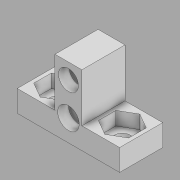
# Autodesk Inventor part: uchwyt_drazki_wersja_2
Saved by Autodesk Inventor 2021 (Build 250183000, 183)
## iProperties
Created: 2022-09-07
Part Number: uchwyt_drazki_wersja_2
Material: Generic
Document SubType Name: Modeling
Designer: agnpi
Density: 1 g/cm^3
Appearance: Default
Author: agnpi
Autodesk Inventor part; units mm, degrees
ref_plane "YZ Plane" through (0, 0, 0) normal (1, 0, 0) x (0, 1, 0)
ref_plane "XZ Plane" through (0, 0, 0) normal (0, 1, 0) x (-1, 0, 0)
ref_plane "XY Plane" through (0, 0, 0) normal (0, 0, 1) x (1, 0, 0)
sketch "Sketch1" plane through (0, 0, 0) normal (0, 1, 0) x (-1, 0, 0)
  line L0 (13.3, 0) -> (-13.3, 0) projected
  line L1 (0, -6.3) -> (0, 6.3) projected
  line L2 (-9.5, 4) -> (9.5, 4)
  line L3 (9.5, 4) -> (9.5, -4)
  line L4 (9.5, -4) -> (-9.5, -4)
  line L5 (-9.5, -4) -> (-9.5, 4)
  line L6 (-9.5, 4) -> (9.5, -4) construction
  line L7 (9.5, 4) -> (-9.5, -4) construction
  point P0 (0, 0)
  dimension "d0" = 19
  dimension "d1" = 8
  constraints: 12 end point, 2 midpoint, 2 parallel, 1 horizontal, 1 perpendicular
  measures "d0" distance of L3.end L4.end
  measures "d1" distance of L2.end L3.end
extrude "Extrusion1" add sketch "Sketch1" along normal blind 13
sketch "Sketch2" plane through (-9.5, 0, 4) normal (0, 0, 1) x (1, 0, 0)
  line L0 (19, 0) -> (0, 0) projected
  line L1 (7, 13) -> (12, 13)
  line L2 (12, 13) -> (12, 0)
  line L3 (12, 0) -> (7, 0)
  line L4 (7, 0) -> (7, 13)
  line L5 (7, 13) -> (12, 0) construction
  line L6 (12, 13) -> (7, 0) construction
  line L7 (0, 13) -> (19, 13) projected
  line L8 (0, 0) -> (0, 13) projected
  line L9 (19, 0) -> (19, 13) projected
  circle A0 centre (9.5, 10.12) radius 1.85
  circle A1 centre (9.5, 4) radius 2
  point P0 (9.5, 0)
  point P1 (9.5, 6.5)
  dimension "d6" = 7
  dimension "d7" = 3.7
  dimension "d8" = 4
  dimension "d9" = 2.5
  dimension "d10" = 2.5
  dimension "d11" = 2
  dimension "d12" = 6.12
  dimension "d19" = 2.5
  constraints: 12 end point, 2 centre point, 2 midpoint, 2 parallel, 1 collinear, 1 horizontal, 1 perpendicular, 1 point on line
  measures "d6" distance between parallel lines of L9 L2
  measures "d7" diameter of A0
  measures "d8" diameter of A1
  measures "d9" distance from line of L2 A0.centre
  measures "d10" distance from line of L2 A1.centre
  measures "d11" distance edge to line of A1 L0
  measures "d12" distance of A0.centre A1.centre
  measures "d19" distance from line of L4 A0.centre
extrude "Extrusion2" cut sketch "Sketch2" against normal blind 2 contours A0 | A1
sketch "Sketch3" plane through (0, 13, 0) normal (0, 1, 0) x (1, 0, 0)
  line L0 (-9.5, -4) -> (9.5, -4) projected
  line L1 (2.5, -4) -> (2.5, 4)
  line L2 (9.5, 4) -> (-9.5, 4) projected
  line L3 (9.5, -4) -> (9.5, 4) projected
  point P0 (0, 0)
  dimension "d15" = 7
  constraints: 2 end point, 2 point on line, 1 parallel
  measures "d15" distance between parallel lines of L3 L1
extrude "Extrusion3" cut sketch "Sketch3" against normal blind 9
sketch "Sketch4" plane through (0, 4, 0) normal (0, 1, 0) x (1, 0, 0)
  line L0 (6, -3.25) -> (3.1854, -1.625)
  line L1 (3.1854, -1.625) -> (3.1854, 1.625)
  line L2 (3.1854, 1.625) -> (6, 3.25)
  line L3 (6, 3.25) -> (8.8146, 1.625)
  line L4 (8.8146, 1.625) -> (8.8146, -1.625)
  line L5 (8.8146, -1.625) -> (6, -3.25)
  line L6 (9.5, -4) -> (2.5, -4) projected
  line L7 (9.5, 4) -> (9.5, -4) projected
  line L8 (2.5, 4) -> (9.5, 4) projected
  point P0 (0, 0)
  point P1 (6, 0)
  dimension "d18" = 6.5
  dimension "d23" = 3.5
  dimension "d24" = 4
  dimension "d32" = 5.6292
  dimension "d33" = 6.5
  constraints: 12 end point, 1 parallel, 13 other
  measures "d18" distance of L0.end L3.end
  measures "d23" distance from line of L7 point (6, 0)
  measures "d24" distance from line of L8 point (6, 0)
  measures "d32" distance between parallel lines of L5 L2
  measures "d33" distance of L0.start L2.end
sketch "Sketch7" plane through (0, 13, 0) normal (0, 1, 0) x (1, 0, 0)
  line L0 (-9.5, -4) -> (2.5, -4) projected
  line L1 (-2.5, -4) -> (-2.5, 4)
  line L2 (2.5, 4) -> (-9.5, 4) projected
  line L3 (-9.5, 4) -> (-9.5, -4) projected
  line L4 (-2.5, -4) -> (-9.5, -4)
  line L5 (-9.5, 4) -> (-2.5, 4)
  point P0 (0, 0)
  dimension "d25" = 7
  constraints: 6 end point, 2 point on line, 1 collinear, 1 parallel, 1 perpendicular
  measures "d25" distance between parallel lines of L3 L1
extrude "Extrusion5" cut sketch "Sketch7" against normal blind 9
sketch "Sketch8" plane through (0, 4, 0) normal (0, 1, 0) x (1, 0, 0)
  line L0 (-3.1854, -1.625) -> (-6, -3.25)
  line L1 (-6, -3.25) -> (-8.8146, -1.625)
  line L2 (-8.8146, -1.625) -> (-8.8146, 1.625)
  line L3 (-8.8146, 1.625) -> (-6, 3.25)
  line L4 (-6, 3.25) -> (-3.1854, 1.625)
  line L5 (-3.1854, 1.625) -> (-3.1854, -1.625)
  line L6 (-2.5, 4) -> (-2.5, -4) projected
  line L7 (-9.5, -4) -> (-9.5, 4) projected
  line L8 (-9.5, 4) -> (-2.5, 4) projected
  point P0 (0, 0)
  point P1 (-6, 0)
  dimension "d28" = 6.5
  dimension "d30" = 3.5
  dimension "d31" = 4
  dimension "d34" = 5.6292
  constraints: 12 end point, 1 parallel, 13 other
  measures "d28" distance of L0.end L3.end
  measures "d30" distance from line of L7 point (-6, 0)
  measures "d31" distance from line of L8 point (-6, 0)
  measures "d34" distance between parallel lines of L0 L3
sketch "Sketch9" plane through (0, 4, 0) normal (0, 1, 0) x (1, 0, 0)
  circle A0 centre (-6, 0) radius 1.5
  line L0 (-2.5, -4) -> (-9.5, -4) projected
  line L1 (-2.5, 4) -> (-2.5, -4) projected
  point P0 (0, 0)
  dimension "d35" = 3
  dimension "d36" = 4
  dimension "d37" = 3.5
  constraints: 1 centre point
  measures "d35" diameter of A0
  measures "d36" distance from line of L0 A0.centre
  measures "d37" distance from line of L1 A0.centre
extrude "Extrusion6" cut sketch "Sketch4" against normal blind 2.5
sketch "Sketch10" plane through (0, 1.5, 0) normal (0, 1, 0) x (1, 0, 0)
  circle A0 centre (6, 0) radius 1.5
  line L0 (9.5, -4) -> (2.5, -4) projected
  line L1 (9.5, 4) -> (9.5, -4) projected
  point P0 (0, 0)
  dimension "d40" = 3
  dimension "d41" = 4
  dimension "d42" = 3.5
  constraints: 1 centre point
  measures "d40" diameter of A0
  measures "d41" distance from line of L0 A0.centre
  measures "d42" distance from line of L1 A0.centre
extrude "Extrusion7" cut sketch "Sketch10" against normal through all
extrude "Extrusion8" cut sketch "Sketch8" against normal blind 2.5
extrude "Extrusion9" cut sketch "Sketch9" against normal through all
body "Solid1"
